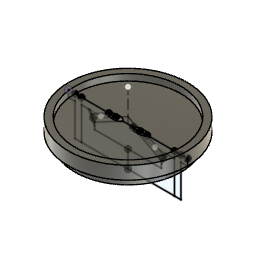
openobs_endcap_angledtxrx_itai (Autodesk Fusion 360 design; units mm, degrees)
Autodesk Fusion 360 part; units mm, degrees
sketch "Sketch10" plane through (0, 0, 0) normal (0, 1, 0) x (1, 0, 0)
  line L0 (0, 0) -> (0, 3)
  line L1 (0, 3) -> (3, 3)
  line L2 (3, 3) -> (3, 18)
  line L3 (3, 18) -> (6, 18)
  line L4 (6, 18) -> (6, 3)
  line L5 (6, 3) -> (10, 3)
  line L6 (10, 3) -> (10.6607, 4.2427)
  line L7 (10, 3) -> (15, 3) construction
  line L8 (10.6607, 4.2427) -> (18.64, 0)
  line L9 (10.6607, 4.2427) -> (12.0691, 6.8915)
  line L10 (0, 0) -> (18.64, 0)
  line L11 (12.0691, 6.8915) -> (25.0302, 0)
  line L12 (25.0302, 0) -> (30, 0)
  line L13 (27.5151, 0) -> (27.5151, -15) construction
  line L14 (12.0691, 6.8915) -> (12.0691, 9.8915)
  line L15 (45.0302, 3) -> (44.3694, 4.2427)
  line L16 (49.0302, 3) -> (45.0302, 3)
  line L17 (55.0302, 0) -> (36.3902, 0)
  line L18 (45.0302, 3) -> (40.0302, 3) construction
  line L19 (44.3694, 4.2427) -> (42.961, 6.8915)
  line L20 (42.961, 6.8915) -> (30, 0)
  line L21 (52.0302, 3) -> (52.0302, 18)
  line L22 (49.0302, 18) -> (49.0302, 3)
  line L23 (55.0302, 3) -> (52.0302, 3)
  line L24 (55.0302, 0) -> (55.0302, 3)
  line L25 (42.961, 6.8915) -> (42.961, 9.8915)
  line L26 (44.3694, 4.2427) -> (36.3902, 0)
  line L27 (52.0302, 18) -> (49.0302, 18)
  line L28 (12.0691, 9.8915) -> (42.961, 9.8915)
  line L29 (42.961, 8.3915) -> (45.8277, 3)
  line L30 (12.0691, 8.3915) -> (9.2024, 3)
  line L31 (52.0302, 3) -> (52.0302, 0) construction
  line L32 (49.0302, 3) -> (49.0302, 0) construction
  line L33 (6, 3) -> (6, 0) construction
  line L34 (3, 3) -> (3, 0) construction
  line L35 (18.64, 0) -> (25.0302, 0) construction
  line L36 (30, 0) -> (36.3902, 0) construction
  line L37 (6, 18) -> (49.0302, 18)
  line L38 (27.5151, 9.8915) -> (27.5151, 18)
  line L39 (43.6652, 5.5671) -> (27.5151, -3.0201) construction
  line L40 (27.5151, -3.0201) -> (11.3649, 5.5671) construction
  point P0 (55.0302, 0)
  point P1 (52.0302, 0)
  point P2 (49.0302, 0)
  point P3 (6, 0)
  point P4 (3, 0)
  point P5 (36.3902, 0)
  point P6 (18.64, 0)
  point P7 (11.3649, 5.5671)
  point P8 (21.8351, 0)
  point P9 (33.1951, 0)
  point P10 (43.6652, 5.5671)
  point P11 (27.5151, 9.8915)
  point P12 (27.5151, 18)
  dimension "d33" = 62
  dimension "d64" = 124
  dimension "d65" = 3
  dimension "d66" = 3
  dimension "d67" = 3
  dimension "d68" = 18.64
  dimension "d69" = 14.6793
  dimension "d70" = 3
  dimension "d71" = 3
  dimension "d72" = 18.2912
  dimension "d73" = 4
  dimension "d74" = 15
  dimension "d75" = 15
  constraint coincident L0.start L10.start
  constraint perpendicular L1 L2
  constraint perpendicular L2 L3
  constraint perpendicular L3 L4
  constraint perpendicular L4 L5
  constraint horizontal L7
  constraint perpendicular L6 L8
  constraint perpendicular L8 L9
  constraint perpendicular L0 L10
  constraint perpendicular L9 L11
  constraint parallel L10 L12
  constraint midpoint L12 L13.start
  constraint perpendicular L12 L13
  constraint vertical L14
  constraint symmetric L0.start L13 L17.start
  constraint symmetric L0.start L13 P0
  constraint symmetric L0.end L13 L23.start
  constraint symmetric L1.end L13 L21.start
  constraint symmetric L2.end L13 L21.end
  constraint symmetric L3.end L13 L22.start
  constraint symmetric L4.end L13 L16.start
  constraint symmetric L5.end L13 L15.start
  constraint symmetric L6.end L13 L15.end
  constraint symmetric L7.end L13 L18.end
  constraint symmetric P6 L13 P5
  constraint symmetric L9.end L13 L19.end
  constraint symmetric L11.end L13 L12.end
  constraint symmetric L13 L14.end L25.end
  constraint perpendicular L25 L28
  constraint midpoint L25 L29.start
  constraint coincident L16 L29.end
  constraint parallel L19 L29
  constraint midpoint L14 L30.start
  constraint coincident L5 L30.end
  constraint parallel L9 L30
  constraint coincident L17 P1
  constraint perpendicular L17 L31
  constraint coincident L17 P2
  constraint perpendicular L17 L32
  constraint coincident L10 P3
  constraint perpendicular L10 L33
  constraint coincident L10 P4
  constraint perpendicular L10 L34
  constraint coincident P1 L31.end
  constraint coincident P2 L32.end
  constraint coincident P3 L33.end
  constraint coincident P4 L34.end
  constraint coincident P5 L17.end
  constraint coincident P6 L8.end
  constraint midpoint L9 P7
  constraint parallel L12 L35
  constraint midpoint L35 P8
  constraint midpoint L36 P9
  constraint midpoint L19 P10
  constraint midpoint L28 P11
  constraint perpendicular L22 L37
  constraint midpoint L37 P12
  constraint coincident P11 L38.start
  constraint coincident P12 L38.end
  constraint perpendicular L37 L38
  constraint coincident P10 L39.start
  constraint coincident L13 L39.end
  constraint perpendicular L19 L39
  constraint coincident P7 L40.end
  measures "d33" angle of L6 L7
  measures "d64" angle of L39 L40
  measures "d65" distance of L23.start P0
  measures "d66" distance of L21.end L22.start
  measures "d67" distance of L2.end L3.end
  measures "d68" distance of P0 P5
  measures "d69" distance of L12.end L19.end
  measures "d70" distance of L25.end L19.end
  measures "d71" distance of L15.end L19.end
  measures "d72" distance of P10 L39.end
  measures "d73" distance of L15.start L16.start
  measures "d74" distance of L21.start L21.end
  measures "d75" distance of L16.start L22.start
sketch "Sketch12" plane through (0, 0, 0) normal (0, 1, 0) x (1, 0, 0)
  line L0 (11.3649, 5.5671) -> (21.8351, 0)
  point P0 (11.3649, 5.5671)
  point P1 (21.8351, 0)
  constraint coincident P0 L0.start
  constraint coincident P1 L0.end
ref_plane "WorkPlane1" through (16.6, 0, -2.7835) normal (0.882948, 0, 0.469472) x (0, 1, 0)
sketch "Sketch17" plane through (16.6, 0, -2.7835) normal (0.882948, 0, 0.469472) x (0, 1, 0)
sketch "Sketch13" plane through (16.6, 0, -2.7835) normal (0.882948, 0, 0.469472) x (0, 1, 0)
  circle A0 centre (0, 0) radius 1.5
  dimension "d41" = 3
  constraint coincident A0.centre origin
  measures "d41" diameter of A0
sketch "Sketch14" plane through (0, 0, 0) normal (0, 1, 0) x (1, 0, 0)
  line L0 (33.1951, 0) -> (43.6652, 5.5671)
  point P0 (33.1951, 0)
  point P1 (43.6652, 5.5671)
  constraint coincident P0 L0.start
  constraint coincident P1 L0.end
ref_plane "WorkPlane2" through (38.4302, 0, -2.7835) normal (0.882948, 0, -0.469472) x (0, 1, 0)
sketch "Sketch15" plane through (38.4302, 0, -2.7835) normal (0.882948, 0, -0.469472) x (0, 1, 0)
  circle A0 centre (0, 0) radius 1.5
  dimension "d43" = 3
  constraint coincident A0.centre origin
  measures "d43" diameter of A0
sketch "Sketch11" plane through (0, 0, 0) normal (0, 0, 1) x (1, 0, 0)
  line L0 (18.64, 0) -> (25.03, 0) construction
  line L1 (36.39, 0) -> (30, 0) construction
  ellipse E0 centre (21.835, 0) end of major axis (18.64, 0) minor radius 1.5
  line L2 (25.03, 0) -> (18.64, 0)
  line L3 (21.835, 1.5) -> (21.835, -1.5)
  line L4 (27.515, 0) -> (27.515, 14) construction
  ellipse E1 centre (33.195, 0) end of major axis (36.39, 0) minor radius 1.5
  circle A0 centre (27.5, 0) radius 27.5
  circle A1 centre (27.5, 0) radius 24.5
  circle A2 centre (27.5, 0) radius 21.5
  point P0 (6, 0)
  dimension "d39" = 3
  dimension "d77" = 43
  dimension "d78" = 49
  dimension "d79" = 55
  constraint horizontal L0
  constraint horizontal L1
  constraint midpoint L0 E0.centre
  constraint coincident L0.end E0
  constraint coincident E0 L3.start
  constraint coincident E0 L3.end
  constraint perpendicular L0 L4
  constraint symmetric E0 L4 E1
  constraint coincident origin A0
  measures "d77" diameter of A2
  measures "d78" diameter of A1
  measures "d79" diameter of A0
extrude "Extrude9" add sketch "Sketch11" against normal up to surface (9.8915 mm away) contours E0 L2 L3 | E0 L2 L3 | E0 L2 L3 | E0 L2 L3 | E1 | A2
extrude "Extrude10" add sketch "Sketch11" against normal blind 7 contours A1
extrude "Extrude11" add sketch "Sketch11" along normal blind 3 and the other way blind 3 contours A0
revolve "Revolve1" cut sketch "Sketch10" angle 360 about axis through (27.5151, 0, 0) along (0, 0, 1) contours L4 L5 L14 L28 L30 L37 L38
revolve "Revolve2" cut sketch "Sketch10" angle 360 about axis through (27.5151, 0, 0) along (0, 0, 1) contours L5 L6 L9 L14 L30 | L4 L5 L14 L28 L30 L37 L38
extrude "Extrude12" cut sketch "Sketch13" along normal through all and the other way up to surface (5.9291 mm away)
extrude "Extrude13" cut sketch "Sketch15" along normal up to surface (5.9291 mm away) and the other way through all
sketch "Sketch16" plane through (0, 0, -9.8915) normal (0, 0, -1) x (1, 0, 0)
  circle A0 centre (27.5151, 0) radius 15.4459
  circle A1 centre (27.5151, 0) radius 13
  dimension "d61" = 26
  constraint concentric A0 A1
  measures "d61" diameter of A1
extrude "Extrude14" cut sketch "Sketch16" against normal blind 2.5 contours A1
sketch "Sketch18" plane through (16.6, 0, -2.7835) normal (0.882948, 0, 0.469472) x (0, 1, 0)
ref_plane "WorkPlane3" through (11.3649, 0, -5.5671) normal (0.882948, 0, 0.469472) x (0, 1, 0)
ref_plane "WorkPlane4" through (43.6652, 0, -5.5671) normal (0.882948, 0, -0.469472) x (0, 1, 0)
